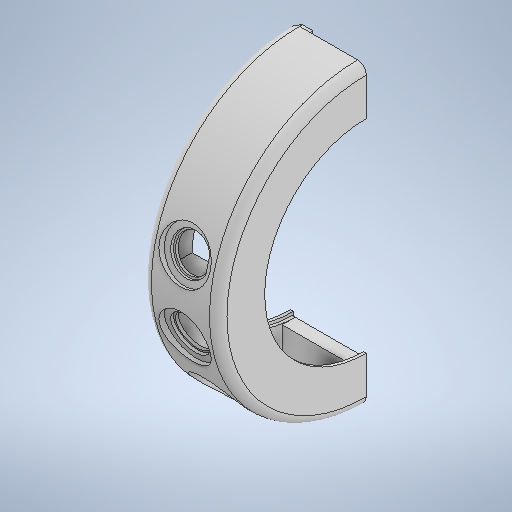
# Autodesk Inventor part: Upper_Part
Saved by Autodesk Inventor 2025.2 (Build 292293000, 293)
## iProperties
Created: 2025-04-17
Part Number: Upper_Part
Material: Generic
Document SubType Name: Modeling
Designer: Andreas
Density: 1 g/cm^3
Appearance: Default
Author: Andreas
Autodesk Inventor part; units mm, degrees
ref_plane "YZ Plane" through (0, 0, 0) normal (1, 0, 0) x (0, 1, 0)
ref_plane "XZ Plane" through (0, 0, 0) normal (0, 1, 0) x (-1, 0, 0)
ref_plane "XY Plane" through (0, 0, 0) normal (0, 0, 1) x (1, 0, 0)
sketch "Sketch1" plane through (0, 0, 0) normal (0, 0, 1) x (1, 0, 0)
  line L0 (0, 0) -> (7.2339, 0)
  line L1 (2, 48) -> (2, 36)
  line L2 (2, 36) -> (1, 36)
  line L3 (1, 36) -> (1, 35)
  line L4 (1, 35) -> (0, 35)
  line L5 (0, 35) -> (0, 51)
  line L6 (0, 51) -> (26, 51)
  line L7 (26, 51) -> (26, 35)
  line L8 (26, 35) -> (25, 35)
  line L9 (25, 35) -> (25, 36)
  line L10 (25, 36) -> (24, 36)
  line L11 (24, 36) -> (24, 48)
  line L12 (24, 48) -> (2, 48)
  dimension "d0" = 1
  dimension "d1" = 26
  dimension "d2" = 102
  dimension "d3" = 3
  dimension "d20" = 70
  constraints: 26 end point, 9 perpendicular, 4 equal length, 4 point on line, 1 horizontal, 1 vertical, 1 vertical alignment
  measures "d0" distance of L3.end L4.end
  measures "d1" distance between parallel lines of L7 L5
  measures "d2" diameter of L6 L0
  measures "d3" distance between parallel lines of L6 L12
  measures "d20" diameter of L4 L0
revolve "Revolution1" add sketch "Sketch1" angle 180 about axis through (0, 0, 0) along (1, 0, 0)
sketch "Sketch2" plane through (26, 35, 0) normal (1, 0, 0) x (0, 0, -1)
  line L0 (0, -35) -> (-17.443, -82.9243)
  arc A0 (0, 16) -> (0, -86) centre (0, -35) ccw projected
  line L1 (0, -70) -> (0, -86) projected
  dimension "d6" = 20
  constraints: 2 end point, 1 point on circle
  measures "d6" angle of L1 L0
ref_plane "Work Plane1" through (26, -47.9243, 17.443) normal (0, -0.9396926, 0.3420201) x (1, 0, 0)
sketch "Sketch5" plane through (26, -47.9243, 17.443) normal (0, -0.9396926, 0.3420201) x (1, 0, 0)
  circle A0 centre (-13, 0) radius 8.75
  line L0 (0, -17.443) -> (-26, -17.443) projected
  point P0 (-26, 0)
  point P1 (-13, -17.443)
  dimension "d14" = 17.5
  constraints: 1 centre point, 1 horizontal alignment, 1 midpoint, 1 vertical alignment
  measures "d14" diameter of A0
extrude "Extrusion3" cut sketch "Sketch5" against normal blind 2
sketch "Sketch3" plane through (26, -47.9243, 17.443) normal (0, -0.9396926, 0.3420201) x (1, 0, 0)
  circle A0 centre (-13, 0) radius 6
  line L0 (0, -17.443) -> (-26, -17.443) projected
  point P0 (-26, 0)
  point P1 (-13, -17.443)
  dimension "d7" = 12
  constraints: 1 centre point, 1 horizontal alignment, 1 midpoint, 1 vertical alignment
  measures "d7" diameter of A0
extrude "Extrusion1" cut sketch "Sketch3" against normal blind 10
sketch "Sketch12" plane through (13, -46.0449, 16.759) normal (0, -0.9396926, 0.3420201) x (1, 0, 0)
  circle A0 centre (0, 0) radius 6 projected
  circle A1 centre (0, 0) radius 8.75 projected
  line L0 (-11, -12.3127) -> (-11, 36) projected
  line L1 (11, -12.3127) -> (11, 36) projected
  line L2 (-11, 8.25) -> (11, 8.25)
  line L3 (11, 8.25) -> (11, -8.25)
  line L4 (11, -8.25) -> (-11, -8.25)
  line L5 (-11, -8.25) -> (-11, 8.25)
  point P0 (-11, 12.3127)
  point P1 (11, 12.3127)
  point P2 (11, 0)
  point P3 (11, 8.25)
  point P4 (-11, -8.25)
  dimension "d53" = 16.5
  constraints: 8 end point, 2 parallel, 2 point on line, 1 horizontal, 1 horizontal alignment, 1 midpoint, 1 perpendicular
  measures "d53" distance between parallel lines of L4 L2
extrude "Extrusion8" add sketch "Sketch12" against normal blind 2 contours A1 L4 L2 | A1 L2 L1 L4 | A1 L4 L0 L2
sketch "Sketch4" plane through (26, -46.0449, 16.759) normal (0, -0.9396926, 0.3420201) x (1, 0, 0)
  circle A0 centre (-13, 0) radius 6.65
  line L0 (0, -17.443) -> (-26, -17.443) projected
  line L1 (-7, 2.8675) -> (-7, -2.8675)
  point P0 (-26, 0)
  point P1 (-13, -17.443)
  point P2 (-7, 0)
  dimension "d10" = 13.3
  dimension "d11" = 6
  constraints: 2 end point, 2 midpoint, 2 point on circle, 1 centre point, 1 horizontal alignment, 1 vertical, 1 vertical alignment
  measures "d10" diameter of A0
  measures "d11" distance of A0.centre point (-7, 0)
extrude "Extrusion2" cut sketch "Sketch4" against normal blind 1 contours L1 A0 picked at (-15.4, -1.0435)
pattern_circular "Circular Pattern1" count 4 over 84 about axis through (-10, 0, 0) along (-1, 0, 0) of "Extrusion3", "Extrusion1", "Extrusion2", "Extrusion8"
fillet "Fillet1" radius 3 2 edges at (26, 0, 51) (0, 0, 51)
sketch "Sketch6" plane through (24, -48, 0) normal (0, 0, -1) x (-1, 0, 0)
  line L0 (0, 0) -> (0, 12) projected
  line L1 (23, 12) -> (22, 12) projected
  line L2 (0, 0) -> (22, 0)
  line L3 (22, 0) -> (22, 12)
  line L4 (22, 12) -> (0, 12)
  line L5 (0, 12) -> (0, 0)
  point P0 (24, 48)
  point P1 (0, 12)
  constraints: 8 end point, 2 parallel, 1 horizontal, 1 perpendicular
extrude "Extrusion4" add sketch "Sketch6" against normal blind 5
sketch "Sketch7" plane through (1, -35, 0) normal (0, 0, -1) x (-1, 0, 0)
  line L0 (1, -13) -> (1, 0) projected
  arc A0 (-2, -16) -> (1, -13) centre (-2, -13) ccw projected
  line L1 (-22, -16) -> (-2, -16) projected
  arc A1 (-25, -13) -> (-22, -16) centre (-22, -13) ccw projected
  line L2 (-25, 0) -> (-25, -13) projected
  line L3 (0, 0) -> (0, -13)
  arc A2 (-2, -15) -> (0, -13) centre (-2, -13) ccw
  line L4 (-2, -15) -> (-22, -15)
  arc A3 (-24, -13) -> (-22, -15) centre (-22, -13) ccw
  line L5 (-24, -13) -> (-24, 0)
  line L6 (0, -0.4915) -> (-24, -0.4915)
  dimension "d24" = 1
  constraints: 8 end point, 4 point on circle, 2 centre point, 2 point on line, 1 perpendicular, 4 other
  measures "d24" distance between parallel lines of L2 L5
extrude "Extrusion5" cut sketch "Sketch7" against normal blind 0.5
sketch "Sketch8" plane through (1, -35, 0.5) normal (0, 0, -1) x (-1, 0, 0)
  line L0 (-23, -1) -> (-1, -1) projected
  point P0 (1, 35)
  point P1 (-12, -10)
  point P2 (-12, -1)
  dimension "d34" = 45
  constraints: 1 midpoint, 1 vertical alignment
  measures "d34" vertical distance of point (1, 35) point (-12, -10)
hole "Hole1" at (13, -45, 0.5) direction (0, 0, 1) diameter 3.8 depth 4.5 tip angle 118
mirror "Mirror1" about plane through (0, 0, 0) normal (0, 1, 0) of "Extrusion4", "Extrusion5", "Hole1"
sketch "Sketch9" plane through (24, 36, 0.5) normal (0, 0, -1) x (-1, 0, 0)
  line L0 (1, 15) -> (21, 15) projected
  line L1 (24, 12) -> (24, -1) projected
  point P0 (24, -36)
  point P1 (19.5, 9)
  dimension "d42" = 6
  dimension "d43" = 4.5
  measures "d42" distance from line of point (19.5, 9) L0
  measures "d43" distance from line of L1 point (19.5, 9)
hole "Hole2" at (4.5, 45, 0.5) direction (0, 0, 1) diameter 4.2 depth 8 tip angle 118
sketch "Sketch10" plane through (24, 36, 0.5) normal (0, 0, -1) x (-1, 0, 0)
  line L0 (21.6, 9) -> (17.4, 9)
  line L1 (17.4, 9) -> (17.4, 0)
  line L2 (17.4, 0) -> (21.6, 0)
  line L3 (21.6, 0) -> (21.6, 9)
  line L4 (22, 0) -> (0, 0) projected
  circle A0 centre (19.5, 9) radius 2.1 projected
  point P0 (24, -36)
  constraints: 8 end point, 2 parallel, 2 tangent, 1 horizontal, 1 perpendicular, 1 point on circle, 1 point on line
extrude "Extrusion6" cut sketch "Sketch10" against normal blind 5 contours A0 L0 | L3 L2 L1 A0 picked at (19.4156, 8.3051)
ref_plane "Work Plane3" through (13, 0, 51) normal (0, 0, -1) x (-1, 0, 0)
ref_plane "Work Plane6" through (13, 0, 49) normal (0, 0, -1) x (-1, 0, 0)
sketch "Sketch11" plane through (24, 0, 49) normal (0, 0, -1) x (-1, 0, 0)
  line L0 (22, 1) -> (0, 1)
  line L1 (0, 1) -> (0, -1)
  line L2 (0, -1) -> (22, -1)
  line L3 (22, -1) -> (22, 1)
  circle A0 centre (11, 0) radius 1.9
  line L4 (11, -1) -> (11, 1) construction
  circle A1 centre (11, 0) radius 3
  line L5 (0, 35.9965) -> (0, -35.9965) projected
  line L6 (22, 35.9965) -> (22, -35.9965) projected
  point P0 (8.1716, -1)
  point P1 (13.8284, -1)
  point P2 (13.8284, 1)
  point P3 (8.1716, 1)
  point P4 (22, 0)
  point P5 (24, 0)
  dimension "d46" = 2
  dimension "d47" = 3.8
  dimension "d48" = 6
  constraints: 10 end point, 4 midpoint, 2 centre point, 2 coincident, 2 parallel, 2 point on line, 1 horizontal, 1 horizontal alignment, 1 perpendicular
  measures "d46" distance of L0.end L1.end
  measures "d47" diameter of A0
  measures "d48" diameter of A1
extrude "Extrusion7" add sketch "Sketch11" along normal up to surface (13 mm away) contours L3 L2 A1 L0 | A1 L2 A0 L0 | L0 A0 A1 | A1 L2 L1 L0 | L0 A0 L2 A1 | A1 L2 A0
sketch "Sketch13" plane through (23, 51, 0) normal (0, 0, -1) x (-1, 0, 0)
  arc A0 (20.6, -6) -> (16.4, -6) centre (18.5, -6) ccw projected
  line L0 (20.6, -6) -> (16.4, -6)
  line L1 (16.4, -6) -> (16.4, 0)
  line L2 (16.4, 0) -> (20.6, 0)
  line L3 (20.6, 0) -> (20.6, -6)
  line L4 (0, 0) -> (20, 0) projected
  arc A1 (23, -3) -> (20, 0) centre (20, -3) ccw projected
  line L5 (0, -1) -> (20, -1) projected
  arc A2 (22, -3) -> (20, -1) centre (20, -3) ccw projected
  point P0 (23, -51)
  point P1 (20.6, -1.0921)
  point P2 (16.4, -1)
  point P3 (20.6, -0.0606)
  constraints: 8 end point, 2 parallel, 1 horizontal, 1 perpendicular, 1 point on line
extrude "Extrusion9" add sketch "Sketch13" against normal blind 2 contours A0 L1 L5 A2 L3
extrude "Extrusion10" add sketch "Sketch13" along normal blind 1 contours A0 L1 L5 A2 L3 | A2 L5 L1 L2 A1 L3
equation "\"d49\" = d48"
body "Solid1"
